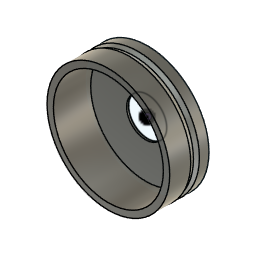
LW_AS_39_1200 (Autodesk Fusion 360 design; units mm, degrees)
Autodesk Fusion 360 part; units mm, degrees
sketch "Sketch1" plane through (0, 0, 0) normal (0, 0, 1) x (1, 0, 0)
  line L0 (0, 40.1335) -> (19.25, 40.1335)
  line L1 (19.25, 40.1335) -> (19.25, 37.1335)
  line L2 (19.25, 37.1335) -> (18.7517, 35.7658)
  line L3 (18.7517, 35.7658) -> (19.2466, 34.4335)
  line L4 (19.2466, 34.4335) -> (19.2466, 27.8335)
  line L5 (19.2466, 27.8335) -> (17.2466, 27.8335)
  line L6 (17.2466, 27.8335) -> (17.2466, 39.5335)
  line L7 (17.2466, 39.5335) -> (0, 39.5335)
  line L8 (0, 39.5335) -> (0, 40.1335)
  dimension "d19" = 19.25
  dimension "d20" = 3
  dimension "d21" = 2.7
  dimension "d22" = 6.6
  dimension "d25" = 2
  dimension "d26" = 11.7
  constraint horizontal L0
  constraint perpendicular L0 L1
  constraint parallel L1 L4
  constraint perpendicular L4 L5
  constraint perpendicular L5 L6
  constraint perpendicular L6 L7
  constraint perpendicular L0 L8
  measures "d19" distance of L0.start L0.end
  measures "d20" distance of L0.end L1.end
  measures "d21" distance of L1.end L3.end
  measures "d22" distance of L3.end L4.end
  measures "d25" distance of L4.end L5.end
  measures "d26" distance of L5.end L6.end
revolve "Revolve1" add sketch "Sketch1" angle 360 about axis through (0, 39.5335, 0) along (0, 1, 0)
sketch "Sketch3" plane through (0, 40.1335, 0) normal (0, 1, 0) x (-1, 0, 0)
  circle A0 centre (0, 0) radius 19.25
  circle A1 centre (0, 0) radius 6
  dimension "d27" = 12
  constraint coincident A0.centre A1.centre
  measures "d27" diameter of A1
extrude "Extrude2" cut sketch "Sketch3" against normal blind 3 contours A1
